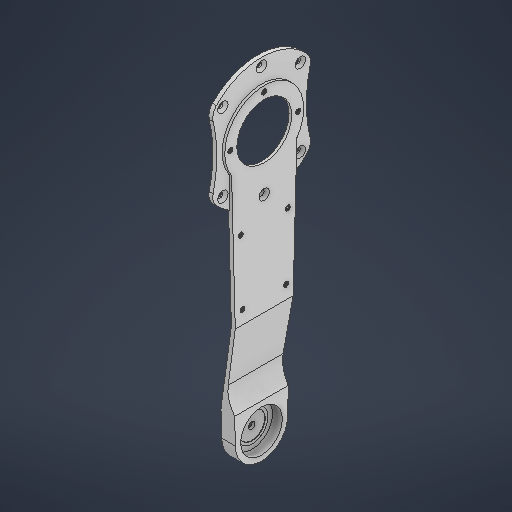
# Autodesk Inventor part: upperleg_gear_side
Saved by Autodesk Inventor 2026 (Build 300175000, 175)
## iProperties
Created: 2025-07-13
Part Number: upperleg_gear_side
Material: Generic
Document SubType Name: Modeling
Designer: User
Density: 1 g/cm^3
Appearance: Default
Author: User
Autodesk Inventor part; units mm, degrees
ref_plane "YZ Plane" through (0, 0, 0) normal (1, 0, 0) x (0, 1, 0)
ref_plane "XZ Plane" through (0, 0, 0) normal (0, 1, 0) x (-1, 0, 0)
sketch "Sketch1" plane through (0, 0, 0) normal (1, 0, 0) x (0, 1, 0)
  circle A0 centre (0, 0) radius 20.5
  constraints: 1 centre point
extrude "Extrusion1" add sketch "Sketch1" along normal blind 3
sketch "Sketch5" plane through (3, 0, 0) normal (1, 0, 0) x (0, 0, -1)
  arc A0 (29.8504, -2.9925) -> (-29.8504, -2.9925) centre (0, 0) ccw construction
  line L0 (30, -200) -> (30, 0) construction
  line L1 (30, -200) -> (20, -200) construction
  line L2 (-30, -200) -> (-20, -200) construction
  circle A1 centre (0, 0) radius 25 construction
  circle A2 centre (0, 0) radius 20.5 projected
  line L3 (0, 0) -> (0, -200) construction
  line L4 (-20, -200) -> (0, -200)
  line L5 (0, -200) -> (20, -200)
  line L6 (-25, 0) -> (-25, -42.4232) construction
  line L7 (25, 0) -> (25, -46.2259) construction
  arc A3 (25, -16.5831) -> (-25, -16.5831) centre (0, 0) ccw
  line L8 (-25, -16.5831) -> (-20, -200)
  line L9 (20, -200) -> (25, -16.5831)
  dimension "d41" = 60
  dimension "d44" = 10
  dimension "d45" = 10
  dimension "d113" = 50
  dimension "d154" = 20
  dimension "d155" = 20
  constraints: 20 end point, 9 point on circle, 3 centre point, 3 coincident, 2 horizontal, 2 point on line, 2 tangent, 2 vertical, 1 collinear
  measures "d41" diameter of A0
  measures "d44" distance of L2.start L2.end
  measures "d45" distance of L1.end L0.start
  measures "d113" diameter of A1
  measures "d154" distance of L2.end L3.end
  measures "d155" distance of L3.end L1.end
extrude "Extrusion3" add sketch "Sketch5" along normal blind 3
sketch "Sketch8" plane through (6, 0, 0) normal (1, 0, 0) x (0, 0, -1)
  line L0 (-20, -200) -> (20, -200) projected
  line L1 (-20, -200) -> (20, -200) projected
  circle A0 centre (0, -200) radius 20
  point P0 (0, 0)
  point P1 (-16.9963, -200)
  point P2 (16.9963, -200)
  constraints: 1 midpoint, 3 other
extrude "Extrusion6" add sketch "Sketch8" against normal up to surface (3 mm away) contours L0 A0 picked at (0.8036, -206.6181)
sketch "Sketch12" plane through (0, 0, 0) normal (-1, 0, 0) x (0, 0, 1)
  circle A0 centre (0, 0) radius 20.75
  dimension "d93" = 41.5
  constraints: 1 centre point, 1 coincident
  measures "d93" diameter of A0
extrude "Extrusion9" cut sketch "Sketch12" against normal blind 14.7
sketch "Sketch13" plane through (3, 0, 0) normal (-1, 0, 0) x (0, 0, 1)
  circle A0 centre (0, 0) radius 30.25
  dimension "d94" = 60.5
  constraints: 1 centre point, 1 coincident
  measures "d94" diameter of A0
extrude "Extrusion10" add sketch "Sketch13" against normal up to surface (3 mm away)
sketch "Sketch14" plane through (3, 0, 0) normal (-1, 0, 0) x (0, 0, 1)
  circle A0 centre (0, 0) radius 21
  dimension "d97" = 42
  constraints: 1 centre point, 1 coincident
  measures "d97" diameter of A0
extrude "Extrusion11" cut sketch "Sketch14" against normal blind 10
sketch "Sketch15" plane through (3, 0, 0) normal (-1, 0, 0) x (0, 0, 1)
  circle A0 centre (0, 0) radius 21
  circle A1 centre (0, 0) radius 30.25
  circle A2 centre (0, 0) radius 48
  dimension "d100" = 96
  constraints: 3 centre point, 3 coincident
  measures "d100" diameter of A2
extrude "Extrusion12" add sketch "Sketch15" along normal blind 2 contours A2
sketch "Sketch16" plane through (1, 0, 0) normal (-1, 0, 0) x (0, 0, 1)
  circle A0 centre (0, 0) radius 41.9754 construction
  circle A1 centre (0, 41.9754) radius 2
  circle A2 centre (0, 0) radius 41.9754 construction
  circle A3 centre (-29.6811, 29.6811) radius 2
  circle A4 centre (0, 0) radius 41.9754 construction
  circle A5 centre (-41.9754, 0) radius 2
  circle A6 centre (0, 0) radius 41.9754 construction
  circle A7 centre (-29.6811, -29.6811) radius 2
  circle A8 centre (0, 0) radius 41.9754 construction
  circle A9 centre (0, -41.9754) radius 2
  circle A10 centre (0, 0) radius 41.9754 construction
  circle A11 centre (29.6811, -29.6811) radius 2
  circle A12 centre (0, 0) radius 41.9754 construction
  circle A13 centre (41.9754, 0) radius 2
  circle A14 centre (0, 0) radius 41.9754 construction
  circle A15 centre (29.6811, 29.6811) radius 2
  dimension "d103" = 83.9508
  dimension "d104" = 4
  dimension "d107" = 360
  constraints: 8 centre point, 2 horizontal alignment, 2 vertical alignment, 1 coincident, 53 other
  measures "d104" diameter of A1
extrude "Extrusion13" cut sketch "Sketch16" against normal blind 9.9375
sketch "Sketch19" plane through (6, 0, 0) normal (1, 0, 0) x (0, 0, -1)
  arc A0 (24.9873, -17.0499) -> (-24.9873, -17.0499) centre (0, 0) ccw projected
  line L0 (20, -200) -> (24.9873, -17.0499) construction
  arc A1 (-20, -200) -> (20, -200) centre (0, -200) ccw construction
  arc A2 (-15.9999, -199.9574) -> (15.9999, -199.9485) centre (0, -200) ccw construction
  circle A3 centre (0, 26) radius 1.5
  circle A4 centre (26, 0) radius 1.5
  line L1 (0, 0) -> (0, -60) construction
  line L2 (0, -60) -> (0, -110) construction
  circle A5 centre (18, -60) radius 1.5
  circle A6 centre (-18, -60) radius 1.5
  circle A7 centre (-16.637, -110) radius 1.5
  circle A8 centre (16.637, -110) radius 1.5
  circle A9 centre (-26, 0) radius 1.5
  line L3 (20, -200) -> (24.9873, -17.0499) projected
  line L4 (-24.9873, -17.0499) -> (-20, -200) projected
  arc A10 (-15.7499, -199.9455) -> (15.7499, -199.9455) centre (0, -200) ccw
  line L5 (0, 0) -> (26, 0) construction
  line L6 (0, 0) -> (-26, 0) construction
  line L7 (0, 0) -> (0, 26) construction
  line L8 (0, -60) -> (18, -60) construction
  line L9 (0, -60) -> (-18, -60) construction
  line L10 (0, -110) -> (16.637, -110) construction
  line L11 (0, -110) -> (-16.637, -110) construction
  dimension "d115" = 3
  dimension "d116" = 3
  dimension "d117" = 60
  dimension "d118" = 50
  dimension "d119" = 3
  dimension "d120" = 3
  dimension "d121" = 3
  dimension "d122" = 3
  dimension "d125" = 3
  dimension "d159" = 26
  dimension "d160" = 18
  dimension "d161" = 18
  dimension "d162" = 16.637
  dimension "d163" = 16.637
  constraints: 18 end point, 9 centre point, 5 horizontal, 4 point on circle, 2 vertical, 1 coincident, 1 perpendicular, 1 point on line
  measures "d115" diameter of A3
  measures "d116" diameter of A4
  measures "d117" distance of L1.start L1.end
  measures "d118" distance of L1.end L2.end
  measures "d119" diameter of A5
  measures "d120" diameter of A6
  measures "d121" diameter of A7
  measures "d122" diameter of A8
  measures "d125" diameter of A9
  measures "d159" distance of L1.start L6.end
  measures "d160" distance of L1.end L8.end
  measures "d161" distance of L1.end L9.end
  measures "d162" distance of L2.end L11.end
  measures "d163" distance of L2.end L10.end
extrude "Extrusion15" cut sketch "Sketch19" against normal blind 3
sketch "Sketch20" plane through (6, 0, 0) normal (1, 0, 0) x (0, 0, -1)
  circle A0 centre (16.637, -110) radius 1.5 projected
  circle A1 centre (0, 26) radius 1.5 projected
  circle A2 centre (18, -60) radius 1.5 projected
  circle A3 centre (-16.637, -110) radius 1.5 projected
  circle A4 centre (26, 0) radius 1.5 projected
  circle A5 centre (-18, -60) radius 1.5 projected
  circle A6 centre (-26, 0) radius 1.5 projected
  circle A7 centre (0, -41.9754) radius 2 projected
  circle A8 centre (0, 0) radius 21 projected
  arc A9 (-20, -200) -> (20, -200) centre (0, -200) ccw projected
  line L0 (20, -200) -> (24.9873, -17.0499) projected
  arc A10 (24.9873, -17.0499) -> (-24.9873, -17.0499) centre (0, 0) ccw projected
  circle A11 centre (-26, 0) radius 1.5 projected
  circle A12 centre (26, 0) radius 1.5 projected
  circle A13 centre (18, -60) radius 1.5 projected
  circle A14 centre (-18, -60) radius 1.5 projected
  circle A15 centre (-16.637, -110) radius 1.5 projected
  circle A16 centre (16.637, -110) radius 1.5 projected
  circle A17 centre (-16.637, -110) radius 2
  circle A18 centre (16.637, -110) radius 2
  circle A19 centre (18, -60) radius 2
  circle A20 centre (-18, -60) radius 2
  circle A21 centre (26, 0) radius 2
  circle A22 centre (-26, 0) radius 2
  circle A23 centre (0, 26) radius 2
  line L1 (-24.9873, -17.0499) -> (-20, -200) projected
  dimension "d130" = 0.5
  dimension "d131" = 0.5
  dimension "d132" = 0.5
  dimension "d133" = 0.5
  dimension "d134" = 0.5
  dimension "d135" = 0.5
  dimension "d136" = 0.5
  constraints: 7 centre point
  measures "d130" radial gap between concentric circles of A3 A17
  measures "d131" radial gap between concentric circles of A0 A18
  measures "d132" radial gap between concentric circles of A2 A19
  measures "d133" radial gap between concentric circles of A5 A20
  measures "d134" radial gap between concentric circles of A4 A21
  measures "d135" radial gap between concentric circles of A6 A22
  measures "d136" radial gap between concentric circles of A1 A23
extrude "Extrusion16" cut sketch "Sketch20" against normal blind 0.5 contours A17 | A18 | A19 | A20 | A21 | A22 | A23
sketch "Sketch21" plane through (3, 0, 0) normal (1, 0, 0) x (0, 0, -1)
  arc A0 (24.324, -41.3805) -> (-24.324, -41.3805) centre (0, 0) ccw projected
  arc A1 (24.9873, -17.0499) -> (-24.9873, -17.0499) centre (0, 0) ccw projected
  line L0 (-24.0975, -18.2859) -> (-20, -200) projected
  circle A2 centre (-29.6811, -29.6811) radius 2 projected
  circle A3 centre (-41.9754, 0) radius 2 projected
  circle A4 centre (-29.6811, 29.6811) radius 2 projected
  circle A5 centre (0, 41.9754) radius 2 projected
  circle A6 centre (29.6811, 29.6811) radius 2 projected
  circle A7 centre (41.9754, 0) radius 2 projected
  circle A8 centre (29.6811, -29.6811) radius 2 projected
  line L1 (24.324, -41.3805) -> (24.9873, -17.0499) projected
  line L2 (-24.9873, -17.0499) -> (-24.324, -41.3805) projected
  line L3 (24.324, -41.3805) -> (24.9873, -17.0499) projected
  arc A9 (24.9873, -17.0499) -> (-24.9873, -17.0499) centre (0, 0) ccw projected
  point P0 (-23.5669, -41.8163)
extrude "Extrusion17" add sketch "Sketch21" along normal blind 1
sketch "Sketch22" plane through (4, 0, 0) normal (1, 0, 0) x (0, 0, -1)
  arc A0 (24.9873, -17.0499) -> (-24.9873, -17.0499) centre (0, 0) ccw projected
  line L0 (-30.25, 0) -> (-34.25, 0) construction
  circle A1 centre (-134.25, 0) radius 100
  line L1 (0, 0) -> (0, 12.7658) construction
  circle A2 centre (134.25, 0) radius 100
  point P0 (-24.0975, -18.2859)
  dimension "d146" = 200
  dimension "d145" = 4
  constraints: 4 end point, 1 centre point, 1 horizontal, 1 horizontal alignment, 1 point on circle, 1 symmetric about line, 1 vertical, 3 other
  measures "d145" distance of L0.start L0.end
extrude "Extrusion18" cut sketch "Sketch22" against normal blind 8.9375
chamfer "Chamfer6" distance 2 angle 45 6 edges at (6, -41.9754, -2) (4, -29.6811, 31.6811) (4, -29.6811, -27.6811) (4, 29.6811, -27.6811) (4, 41.9754, 2) (4, 29.6811, 31.6811)
fillet "Fillet2" radius 10 8 edges at (2, -28.7171, 38.4621) (3.5, -28.7171, 38.4621) (3.5, 28.7171, 38.4621) (2, 28.7171, 38.4621) (3.5, -28.7171, -38.4621) (2, -28.7171, -38.4621) (2, 28.7171, -38.4621) (3.5, 28.7171, -38.4621)
fillet "Fillet3" radius 2 1 edges at (3, -48, 0)
chamfer "Chamfer8" distance 2 angle 45 3 edges at (3, 0, -24.5) (3, 26, 1.5) (3, 0, 27.5)
chamfer "Chamfer9" distance 2 angle 45 4 edges at (3, -60, -16.5) (3, -60, 19.5) (3, -110, -15.137) (3, -110, 18.137)
sketch "Sketch25" plane through (3, 0, 0) normal (-1, 0, 0) x (0, 0, 1)
  arc A0 (-20, -200) -> (20, -200) centre (0, -200) ccw projected
  line L0 (0, -200) -> (0, -120)
  line L1 (-20, -200) -> (-24.2602, -43.72) projected
  line L2 (24.2602, -43.72) -> (20, -200) projected
  line L3 (-22.1808, -120) -> (22.1808, -120)
  point P0 (0, 0)
  dimension "d179" = 80
  constraints: 4 end point, 2 point on line, 1 horizontal, 1 midpoint, 1 vertical
  measures "d179" distance of L0.start L0.end
extrude "Extrusion21" add sketch "Sketch25" along normal blind 9.6
ref_plane "Work Plane1" through (-6.6, -933.6675, 0) normal (0, 0, 1) x (-1, 0, 0)
sketch "Sketch26" plane through (-6.6, -933.6675, 0) normal (0, 0, 1) x (-1, 0, 0)
  line L0 (0, -733.6675) -> (0, -713.6675) projected
  line L1 (0, -713.6675) -> (0, -753.6675) construction
  line L2 (0, -733.6675) -> (0, -813.6675) projected
  line L3 (-9.6, -889.9475) -> (-9.6, -813.6675) projected
  line L4 (0, -753.6675) -> (-9.6, -813.6675)
  line L5 (-9.6, -813.6675) -> (0, -813.6675) projected
  line L6 (-9.6, -813.6675) -> (0, -813.6675)
  line L7 (0, -813.6675) -> (0, -753.6675)
  point P0 (-6.6, -933.6675)
  dimension "d182" = 40
  constraints: 8 end point, 1 collinear, 1 perpendicular, 1 point on line
  measures "d182" distance of L0.end L1.end
extrude "Extrusion22" cut sketch "Sketch26" along normal mid plane 65.3875
chamfer "Chamfer10" distance 1 angle 45 1 edges at (3, 0, -21)
sketch "Sketch31" plane through (-6.6, -933.6675, 0) normal (0, 0, 1) x (-1, 0, 0)
  line L0 (0, -753.6675) -> (-9.6, -813.6675) projected
  line L1 (-3.0382, -753.6675) -> (-12.6, -813.429)
  line L2 (-12.6, -713.6675) -> (0, -713.6675) construction
  line L3 (0, -733.6675) -> (0, -713.6675) construction
  line L4 (0, -753.6675) -> (0, -733.6675) construction
  line L5 (-12.6, -713.6675) -> (-12.6, -753.6675) construction
  line L6 (-12.6, -916.6176) -> (-12.6, -733.6675) construction
  line L7 (0, -733.6675) -> (-12.6, -733.6675) construction
  line L8 (-13.8183, -753.6675) -> (-13.8183, -813.4187)
  line L9 (-13.8183, -813.4187) -> (-12.6, -813.429)
  line L10 (-12.6, -733.6675) -> (-12.6, -916.6176) construction
  line L11 (-13.8183, -753.6675) -> (-3.0382, -753.6675)
  point P0 (-6.6, -933.6675)
  dimension "d205" = 3
  dimension "d206" = 40
  constraints: 10 end point, 2 parallel, 2 point on line, 1 perpendicular
  measures "d205" distance between parallel lines of L0 L1
  measures "d206" distance of L2.start L5.end
extrude "Extrusion27" cut sketch "Sketch31" along normal mid plane 87.3875
sketch "Sketch32" plane through (6, 0, 0) normal (1, 0, 0) x (0, 0, -1)
  arc A0 (-20, -200) -> (20, -200) centre (0, -200) ccw projected
  circle A1 centre (0, -200) radius 16
  point P0 (0, 0)
  dimension "d213" = 32
  constraints: 1 centre point, 1 coincident
  measures "d213" diameter of A1
extrude "Extrusion28" cut sketch "Sketch32" against normal blind 9.6
sketch "Sketch33" plane through (-3.6, -200, 0) normal (1, 0, 0) x (0, 0, -1)
  circle A0 centre (0, 0) radius 16 projected
  circle A1 centre (0, 0) radius 10
  circle A2 centre (0, 0) radius 12
  point P0 (0, 200)
  dimension "d216" = 20
  dimension "d217" = 24
  constraints: 2 centre point, 2 coincident
  measures "d216" diameter of A1
  measures "d217" diameter of A2
extrude "Extrusion29" add sketch "Sketch33" along normal blind 0.5 contours A2
sketch "Sketch34" plane through (6, 0, 0) normal (1, 0, 0) x (0, 0, -1)
  circle A0 centre (0, -200) radius 16 projected
  line L0 (20.5452, -180) -> (-20.5452, -180) projected
  line L1 (-24.9873, -17.0499) -> (-20, -200) projected
  arc A1 (-20, -200) -> (20, -200) centre (0, -200) ccw projected
  line L2 (20, -200) -> (20.5452, -180) projected
  point P0 (0, 0)
extrude "Extrusion30" cut sketch "Sketch34" against normal blind 2.1
fillet "Fillet8" radius 25 1 edges at (-3.5618, -180, 0)
sketch "Sketch35" plane through (-6.6, 0, 0) normal (-1, 0, 0) x (0, 0, 1)
  arc A0 (-20, -200) -> (20, -200) centre (0, -200) ccw projected
  circle A1 centre (0, -200) radius 2.5
  point P0 (0, 0)
  dimension "d223" = 5
  constraints: 1 centre point, 1 coincident
  measures "d223" diameter of A1
extrude "Extrusion31" cut sketch "Sketch35" against normal blind 29.0875
chamfer "Chamfer11" distance 1 angle 45 1 edges at (-6.6, -200, -2.5)
body "Solid1"
